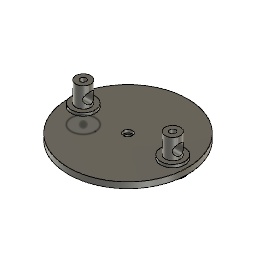
servo-ring (Autodesk Fusion 360 design; units mm, degrees)
part number: 2026-01-12-14-24-57-447
Autodesk Fusion 360 part; units mm, degrees
sketch "outer-circle+hole" plane through (0, 0, 0) normal (0, 0, 1) x (1, 0, 0)
  circle A0 centre (0, 0) radius 20
  circle A1 centre (0, 0) radius 2.5
  circle A2 centre (0, 0) radius 1
  circle A3 centre (0, 0) radius 3.5
  circle A4 centre (0, 0) radius 1.5
  dimension "d1" = 40
  dimension "d2" = 5
  dimension "d3" = 2
  dimension "d4" = 7
  dimension "d11" = 3
  constraint coincident A0.centre A1.centre
  constraint concentric A0 A1
  constraint concentric A0 A2
  constraint concentric A3 A4
  measures "d1" diameter of A0
  measures "d2" diameter of A1
  measures "d3" diameter of A2
  measures "d4" diameter of A3
  measures "d11" diameter of A4
extrude "Extrude1" add sketch "outer-circle+hole" along normal blind 2 contours A0 | A1 | A2 | A3 | A4 makes body 1
extrude "Extrude2" add sketch "outer-circle+hole" against normal blind 3 contours A3 bodies 1
extrude "Extrude3" cut sketch "outer-circle+hole" along normal blind 6 contours A2 bodies 1
sketch "Sketch2" plane through (0, 0, 2) normal (0, 0, 1) x (-1, 0, 0)
  circle A0 centre (0, 0) radius 1
  circle A1 centre (0, 0) radius 20
  circle A2 centre (0, 0) radius 1.5
  dimension "d12" = 3
  constraint coincident A0.centre A1.centre
  measures "d12" diameter of A2
extrude "Extrude4" cut sketch "Sketch2" against normal blind 1 contours A2 bodies 1
sketch "Sketch3" plane through (0, 0, 2) normal (0, 0, 1) x (-1, 0, 0)
  circle A0 centre (0, 0) radius 1.5
  circle A1 centre (0, 0) radius 20
  circle A2 centre (15, 0) radius 3
  circle A3 centre (15, 0) radius 2.5
  circle A4 centre (-15, 0) radius 2.5
  circle A5 centre (-15, 0) radius 3
  dimension "d15" = 6
  dimension "d16" = 5
  dimension "d37" = 15
  dimension "d38" = 6
  dimension "d39" = 5
  dimension "d40" = 15
  constraint concentric A2 A3
  constraint concentric A4 A5
  measures "d15" diameter of A2
  measures "d16" diameter of A3
  measures "d37" distance of A0.centre A2.centre
  measures "d38" diameter of A5
  measures "d39" diameter of A4
  measures "d40" distance of A0.centre A4.centre
extrude "Extrude5" cut sketch "Sketch3" against normal blind 10 contours A2 | A3 bodies 1
extrude "Extrude6" add sketch "Sketch3" along normal blind 18 separate body contours A3 makes body 2
extrude "Extrude7" cut 1 faces at (-14.3115, -0.4694, 20) along direction (0, 0, -1) blind 10 on bodies 2 bodies 2
move_face "MoveFace1" to x (1, 0, 0) y (0, 1, 0) z (0, 0, 1) at (0, 0, -5) 1 faces at (-17.4876, 0.2489, 4.6667) on bodies 2
move_body "Move1" bodies 2 to x (1, 0, 0) y (0, 1, 0) z (0, 0, 1) at (0, 0, -5)
extrude "Extrude8" add 1 faces at (-14.3115, -0.4694, 5) along direction (0, 0, 1) blind 5 on bodies 2 bodies 2
sketch "Sketch5" plane through (0, 0, -3) normal (0, 0, -1) x (1, 0, 0)
  circle A0 centre (-15, 0) radius 2.5
  circle A1 centre (-15, 0) radius 4
  dimension "d26" = 8
  constraint concentric A0 A1
  measures "d26" diameter of A1
extrude "Extrude9" add sketch "Sketch5" against normal blind 1 contours A0 | A1 bodies 2
sketch "Sketch7" plane through (0, 0, 0) normal (1, 0, 0) x (0, 1, 0)
  circle A0 centre (0, 6) radius 1.85
  dimension "d29" = 3.7
  measures "d29" diameter of A0
extrude "Extrude10" cut sketch "Sketch7" against normal blind 32 bodies 2
sketch "Sketch8" plane through (0, 0, 10) normal (0, 0, 1) x (-1, 0, 0)
  circle A0 centre (15, 0) radius 2.5
  circle A1 centre (15, 0) radius 1
  dimension "d32" = 2
  constraint concentric A0 A1
  measures "d32" diameter of A1
extrude "Extrude11" cut sketch "Sketch8" against normal blind 5 contours A1 bodies 2
move_face "MoveFace2" to x (1, 0, 0) y (0, 1, 0) z (0, 0, 1) at (0, 0, 1.5) 3 faces at (-11.5242, 0.3229, -2) (-11.0199, 0.3983, -2.6667) (-14.1687, 1.0424, -3) on bodies 2
extrude "Extrude12" add sketch "Sketch5" along normal blind 1 separate body contours A0 | A1 makes body 3
move_body "Move2" bodies 3 to x (1, 0, 0) y (0, 1, 0) z (0, 0, 1) at (0, 0, 6)
move_body "Move3" bodies 3 to x (1, 0, 0) y (0, 1, 0) z (0, 0, 1) at (0, 0, 0.5)
combine "Combine1" operation add target body 2 tool bodies 3
extrude "Extrude13" cut sketch "Sketch3" against normal blind 10 contours A4 | A5 bodies 1
move_face "MoveFace3" to x (1, 0, 0) y (0, 1, 0) z (0, 0, 1) at (0, 0, 0.25) 3 faces at (-11.0199, 0.3983, -0.8333) (-11.5242, 0.3229, -0.5) (-14.1687, 1.0424, -1.5) on bodies 2
move_face "MoveFace4" to x (1, 0, 0) y (0, 1, 0) z (0, 0, 1) at (0, 0, -0.25) 3 faces at (-11.5242, 0.3229, 3.5) (-11.0199, 0.3983, 3.1667) (-11.5242, 0.3229, 2.5) on bodies 2
copy_body "CopyPasteBodies2" bodies 2 makes body 4
move_body "Move5" bodies 4 to x (1, 0, 0) y (0, 1, 0) z (0, 0, 1) at (30, 0, 0)
sketch "Sketch6" plane through (0, 0, 2) normal (0, 0, 1) x (-1, 0, 0)
sketch "Sketch4" plane through (0, 0, 2) normal (0, 0, 1) x (-1, 0, 0)
  circle A0 centre (15, 0) radius 4
  dimension "d25" = 8
  measures "d25" diameter of A0
named bodies: "Circle"
